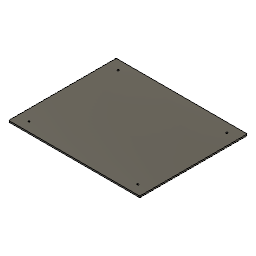
bottom_panel v1 (Autodesk Fusion 360 design; units mm, degrees)
Autodesk Fusion 360 part; units mm, degrees
sketch "Sketch1" plane through (0, 0, 0) normal (0, 0, 1) x (1, 0, 0)
  line L0 (2, 0) -> (278, 0)
  line L1 (280, 2) -> (280, 228)
  line L2 (278, 230) -> (2, 230)
  line L3 (0, 228) -> (0, 2)
  circle A0 centre (24, 210) radius 1.65
  circle A1 centre (256, 210) radius 1.65
  circle A2 centre (24, 20) radius 1.65
  circle A3 centre (256, 20) radius 1.65
  arc A4 (2, 230) -> (0, 228) centre (2, 228) ccw
  arc A5 (280, 228) -> (278, 230) centre (278, 228) ccw
  arc A6 (278, 0) -> (280, 2) centre (278, 2) ccw
  arc A7 (0, 2) -> (2, 0) centre (2, 2) ccw
  point P0 (280, 0)
  point P1 (0, 230)
  dimension "d1" = 280
  dimension "d2" = 230
  dimension "d3" = 3.3
  dimension "d5" = 24
  dimension "d6" = 20
  dimension "d9" = 232
  dimension "d10" = -190
  dimension "d12" = 2
  constraint horizontal L0
  constraint vertical L1
  constraint horizontal L2
  constraint vertical L3
  constraint coincident P1 L2
  constraint coincident P1 L3
  constraint tangent L2 A4
  constraint tangent L3 A4
  constraint tangent L1 A5
  constraint tangent L2 A5
  constraint equal A4 A5
  constraint coincident P0 L0
  constraint coincident P0 L1
  constraint tangent L0 A6
  constraint tangent L1 A6
  constraint equal A4 A6
  constraint coincident origin L0
  constraint coincident origin L3
  constraint tangent L0 A7
  constraint tangent L3 A7
  constraint equal A4 A7
  measures "d1" distance of origin P0
  measures "d2" distance of origin P1
  measures "d3" diameter of A0
  measures "d5" distance of L3 A0.centre
  measures "d6" distance of L2 A0.centre
  measures "d12" radius of A4
extrude "Extrude1" add sketch "Sketch1" along normal blind 3
equation "d3 = hole_width"
equation "hole_width = 3.3 mm"
equation "d9 = 280 mm - ( 24 * 2 ) * 1 mm"
equation "d10 = -( 230 mm - ( 20 * 2 ) * 1 mm )"
equation "outer_rad = 2 mm"
